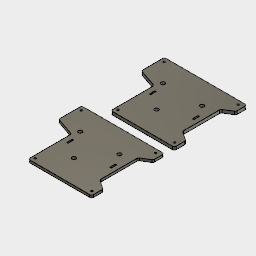
Y_Carriage_v1 (Autodesk Fusion 360 design; units mm, degrees)
Autodesk Fusion 360 part; units mm, degrees
sketch "Sketch1" plane through (0, 0, 0) normal (0, 1, 0) x (1, 0, 0)
  line L0 (-70, 48.432) -> (-70, 17.1623)
  line L1 (-67.9487, 14.3162) -> (-41.8723, 5.6241)
  line L2 (-39.821, 2.7781) -> (-39.821, -60.1467)
  line L3 (-36.821, -63.1467) -> (57.179, -63.1467)
  line L4 (60.179, -60.1467) -> (60.179, -46.7249)
  line L5 (58.8431, -44.2287) -> (46.3359, -35.8906)
  line L6 (45, -33.3944) -> (45, 23.3232)
  line L7 (46.4283, 25.8785) -> (58.5717, 33.3476)
  line L8 (60, 35.9029) -> (60, 48.432)
  line L9 (57, 51.432) -> (-67, 51.432)
  line L10 (-31.8938, -1.3937) -> (-30, -1.3937)
  line L11 (-30, -1.3937) -> (-30, -10)
  line L12 (-30, -10) -> (-31.8938, -10)
  line L13 (-31.8938, -10) -> (-31.8938, -1.3937)
  line L14 (35.7659, -1.3937) -> (37.9138, -1.3937)
  line L15 (37.9138, -1.3937) -> (37.9138, -10)
  line L16 (37.9138, -10) -> (35.7659, -10)
  line L17 (35.7659, -10) -> (35.7659, -1.3937)
  circle A0 centre (-5, -25.8352) radius 3
  circle A1 centre (-35.8854, 15) radius 3
  circle A2 centre (25.6268, 15) radius 3
  circle A3 centre (-35.1495, -56.5239) radius 1.5
  circle A4 centre (54.0379, -56.5239) radius 1.5
  circle A5 centre (52.4619, 45) radius 1.5
  circle A6 centre (-64.0904, 45) radius 1.5
  arc A7 (-67, 51.432) -> (-70, 48.432) centre (-67, 48.432) ccw
  arc A8 (60, 48.432) -> (57, 51.432) centre (57, 48.432) ccw
  arc A9 (58.5717, 33.3476) -> (60, 35.9029) centre (57, 35.9029) ccw
  arc A10 (46.4283, 25.8785) -> (45, 23.3232) centre (48, 23.3232) ccw
  arc A11 (45, -33.3944) -> (46.3359, -35.8906) centre (48, -33.3944) ccw
  arc A12 (60.179, -46.7249) -> (58.8431, -44.2287) centre (57.179, -46.7249) ccw
  arc A13 (57.179, -63.1467) -> (60.179, -60.1467) centre (57.179, -60.1467) ccw
  arc A14 (-39.821, -60.1467) -> (-36.821, -63.1467) centre (-36.821, -60.1467) ccw
  arc A15 (-39.821, 2.7781) -> (-41.8723, 5.6241) centre (-42.821, 2.7781) ccw
  arc A16 (-70, 17.1623) -> (-67.9487, 14.3162) centre (-67, 17.1623) ccw
  dimension "d1" = 6
  dimension "d2" = 6
  dimension "d3" = 6
  dimension "d4" = 3
  dimension "d5" = 3
  dimension "d6" = 3
  dimension "d7" = 3
  dimension "d8" = 3
  measures "d1" diameter of A0
  measures "d2" diameter of A1
  measures "d3" diameter of A2
  measures "d4" diameter of A3
  measures "d5" diameter of A4
  measures "d6" diameter of A5
  measures "d7" diameter of A6
  measures "d8" radius of A7
extrude "Extrude1" add sketch "Sketch1" along normal blind 5 makes body 1
copy_body "CopyPasteBodies1" bodies 1 makes body 2
move_body "Move1" bodies 2 to x (1, 0, 0) y (0, 1, 0) z (0, 0, 1) at (0, 0, 130)
move_face "OffsetFaces1" offset -1 1 faces at (-15.338, 5, 93.7001) on bodies 2
named bodies: "5mm", "4mm"
